Autodesk Fusion 360 part; units mm, degrees
note: some values were not read from the file. Chosen so that the rebuilt part matches the saved one: which bodies a step acts on; a direction. Set by a fixed rule: which sketch regions a step uses.
(part 5 of 5)
sketch "Ear sketch" plane through (0, 0, 0) normal (0, 0, 1) x (1, 0, 0) in component "Stepper bay 28BYJ-48"
  line L0 (-3.4154, 1.0961) -> (0.7978, -2.4393)
  arc A0 (-3.7017, -7.8016) -> (0.7978, -2.4393) centre (-1.4519, -5.1204) ccw
  line L1 (-3.7017, -7.8016) -> (-7.9149, -4.2663)
  arc A1 (-3.4154, 1.0961) -> (-7.9149, -4.2663) centre (-5.6652, -1.5851) ccw
extrude "Ear" add sketch "Ear sketch" along normal blind 7 from surface at 80 bodies 224 in component "Stepper bay 28BYJ-48"
sketch "Ear sketch (1)" plane through (0, 0, 0) normal (0, 0, 1) x (1, 0, 0) in component "Stepper bay 28BYJ-48"
  line L0 (-26.3, 11.1607) -> (-30.5132, 14.696)
  arc A0 (-26.0137, 20.0583) -> (-30.5132, 14.696) centre (-28.2635, 17.3771) ccw
  line L1 (-26.0137, 20.0583) -> (-21.8005, 16.523)
  arc A1 (-26.3, 11.1607) -> (-21.8005, 16.523) centre (-24.0502, 13.8418) ccw
extrude "Ear (1)" add sketch "Ear sketch (1)" along normal blind 7 from surface at 80 bodies 224 in component "Stepper bay 28BYJ-48"
sketch "Wire block sketch" plane through (0, 0, 0) normal (0, 0, 1) x (1, 0, 0) in component "Stepper bay 28BYJ-48"
  line L0 (-9.5224, 23.8435) -> (-12.7364, 20.0132)
  line L1 (-12.7364, 20.0132) -> (-1.5521, 10.6285)
  line L2 (-1.5521, 10.6285) -> (1.6618, 14.4588)
  line L3 (1.6618, 14.4588) -> (-9.5224, 23.8435)
extrude "Wire block" add sketch "Wire block sketch" along normal blind 19 from surface at 68 bodies 224 in component "Stepper bay 28BYJ-48"
component "Tub" placed x (1, 0, 0) y (0, 1, 0) z (0, 0, 1) at (0, 0, 0)
component "Wheel L" placed x (1, 0, 0) y (0, 1, 0) z (0, 0, 1) at (0, 0, 0)
component "Motor L" placed x (1, 0, 0) y (0, 1, 0) z (0, 0, 1) at (0, 0, 0)
component "Wheel R" placed x (1, 0, 0) y (0, 1, 0) z (0, 0, 1) at (0, 0, 0)
component "Motor R" placed x (1, 0, 0) y (0, 1, 0) z (0, 0, 1) at (0, 0, 0)
component "Face plate L" placed x (1, 0, 0) y (0, 1, 0) z (0, 0, 1) at (0, 0, 0)
component "Face plate R" placed x (1, 0, 0) y (0, 1, 0) z (0, 0, 1) at (0, 0, 0)
component "Omni wheel" placed x (1, 0, 0) y (0, 1, 0) z (0, 0, 1) at (0, 0, 0)
component "Omni arm" placed x (1, 0, 0) y (0, 1, 0) z (0, 0, 1) at (0, 0, 0)
component "Omni pins" placed x (1, 0, 0) y (0, 1, 0) z (0, 0, 1) at (0, 0, 0)
component "Omni pivot" placed x (1, 0, 0) y (0, 1, 0) z (0, 0, 1) at (0, 0, 0)
component "Omni spring" placed x (1, 0, 0) y (0, 1, 0) z (0, 0, 1) at (0, 0, 0)
component "Omni adjuster" placed x (1, 0, 0) y (0, 1, 0) z (0, 0, 1) at (0, 0, 0)
component "Rear nub" placed x (1, 0, 0) y (0, 1, 0) z (0, 0, 1) at (0, 0, 0)
component "Bumper L" placed x (1, 0, 0) y (0, 1, 0) z (0, 0, 1) at (0, 0, 0)
component "Bumper switch L" placed x (1, 0, 0) y (0, 1, 0) z (0, 0, 1) at (0, 0, 0)
component "Bumper R" placed x (1, 0, 0) y (0, 1, 0) z (0, 0, 1) at (0, 0, 0)
component "Bumper switch R" placed x (1, 0, 0) y (0, 1, 0) z (0, 0, 1) at (0, 0, 0)
component "Upper frame" placed x (1, 0, 0) y (0, 1, 0) z (0, 0, 1) at (0, 0, 0)
component "ToF F" placed x (1, 0, 0) y (0, 1, 0) z (0, 0, 1) at (0, 0, 0)
component "ToF FL" placed x (1, 0, 0) y (0, 1, 0) z (0, 0, 1) at (0, 0, 0)
component "ToF FR" placed x (1, 0, 0) y (0, 1, 0) z (0, 0, 1) at (0, 0, 0)
component "ToF SFL" placed x (1, 0, 0) y (0, 1, 0) z (0, 0, 1) at (0, 0, 0)
component "ToF SFR" placed x (1, 0, 0) y (0, 1, 0) z (0, 0, 1) at (0, 0, 0)
component "ToF SRL" placed x (1, 0, 0) y (0, 1, 0) z (0, 0, 1) at (0, 0, 0)
component "ToF SRR" placed x (1, 0, 0) y (0, 1, 0) z (0, 0, 1) at (0, 0, 0)
component "ToF RL" placed x (1, 0, 0) y (0, 1, 0) z (0, 0, 1) at (0, 0, 0)
component "ToF RR" placed x (1, 0, 0) y (0, 1, 0) z (0, 0, 1) at (0, 0, 0)
component "Camera L" placed x (1, 0, 0) y (0, 0.34202, 0.939693) z (0, -0.939693, 0.34202) at (3.0712, 87.9464, 93)
component "Camera cage L" placed x (1, 0, 0) y (0, 1, 0) z (0, 0, 1) at (0, 0, 0)
component "Camera R" placed x (-1, 0, 0) y (0, -0.34202, 0.939693) z (0, 0.939693, 0.34202) at (3.0712, -87.9464, 93)
component "Camera cage R" placed x (1, 0, 0) y (0, 1, 0) z (0, 0, 1) at (0, 0, 0)
component "Lid" placed x (1, 0, 0) y (0, 1, 0) z (0, 0, 1) at (0, 0, 0)
component "Handle bar" placed x (1, 0, 0) y (0, 1, 0) z (0, 0, 1) at (0, 0, 0)
component "Victim LED" placed x (1, 0, 0) y (0, 1, 0) z (0, 0, 1) at (0, 0, 0)
component "Start button" placed x (1, 0, 0) y (0, 1, 0) z (0, 0, 1) at (0, 0, 0)
component "Power switch" placed x (1, 0, 0) y (0, 1, 0) z (0, 0, 1) at (0, 0, 0)
component "Status LED 1" placed x (1, 0, 0) y (0, 1, 0) z (0, 0, 1) at (0, 0, 0)
component "Status LED 2" placed x (1, 0, 0) y (0, 1, 0) z (0, 0, 1) at (0, 0, 0)
component "USB-C service socket" placed x (1, 0, 0) y (0, 1, 0) z (0, 0, 1) at (0, 0, 0)
component "Dropper floor" placed x (1, 0, 0) y (0, 1, 0) z (0, 0, 1) at (0, 0, 0)
component "Dropper plate" placed x (1, 0, 0) y (0, 1, 0) z (0, 0, 1) at (0, 0, 0)
component "N20 motor" placed x (1, 0, 0) y (0, 1, 0) z (0, 0, 1) at (0, 0, 0)
component "N20 face plate" placed x (1, 0, 0) y (0, 1, 0) z (0, 0, 1) at (0, 0, 0)
component "Kits" placed x (1, 0, 0) y (0, 1, 0) z (0, 0, 1) at (0, 0, 0)
component "Hopper B left" placed x (1, 0, 0) y (0, 1, 0) z (0, 0, 1) at (0, 0, 0)
component "Chute B left" placed x (1, 0, 0) y (0, 1, 0) z (0, 0, 1) at (0, 0, 0)
component "Hopper A right" placed x (1, 0, 0) y (0, 1, 0) z (0, 0, 1) at (0, 0, 0)
component "Chute A right" placed x (1, 0, 0) y (0, 1, 0) z (0, 0, 1) at (0, 0, 0)
component "GIGA posts" placed x (1, 0, 0) y (0, 1, 0) z (0, 0, 1) at (0, 0, 0)
component "Arduino GIGA R1" placed x (1, 0, 0) y (0, 1, 0) z (0, 0, 1) at (0, 0, 0)
component "Main PCB" placed x (1, 0, 0) y (0, 1, 0) z (0, 0, 1) at (0, 0, 0)
component "Battery" placed x (1, 0, 0) y (0, 1, 0) z (0, 0, 1) at (0, 0, 0)
component "Floor port FP" placed x (1, 0, 0) y (0, 1, 0) z (0, 0, 1) at (0, 0, 0)
component "Silver module SM" placed x (1, 0, 0) y (0, 1, 0) z (0, 0, 1) at (0, 0, 0)
component "Wi-Fi antenna" placed x (1, 0, 0) y (0, 1, 0) z (0, 0, 1) at (0, 0, 0)
component "BNO055 IMU" placed x (1, 0, 0) y (0, 1, 0) z (0, 0, 1) at (0, 0, 0)
component "Stepper bay 28BYJ-48" placed x (1, 0, 0) y (0, 1, 0) z (0, 0, 1) at (0, 0, 0)
named bodies: "Tub shell", "Chute hole tool B left", "Chute hole tool A right", "Cradle prong front L", "Cradle prong rear L", "Cradle prong front R", "Cradle prong rear R", "Wheel L", "Encoder L", "Gearmotor L", "Motor shaft L", "Wheel R", "Encoder R", "Gearmotor R", "Motor shaft R", "Face plate L", "Face plate R", "Omni wheel", "Bearing inboard", "Bearing outboard", "Axle sleeve", "Axle spacer", "Arm bar", "Seat pin", "Spring forward leg", "Axle screw", "Axle screw head", "Axle washer", "Pivot screw", "Pivot screw head", "Stop screw", "Stop screw head", "Pivot tube", "Spring coil", "Spring rear leg", "Spring arbor", "Adjuster screw head", "Adjuster screw", "Rear nub", "Bumper plate L", "Microswitch L", "Bumper plate R", "Microswitch R", "Frame ring", "VL53L0X board F", "QT connector F", "QT connector F (1)", "VL53L0X chip F", "M2.5 screw heads F 1", "M2.5 screw heads F 2", "M2.5 screw shafts F 1", "M2.5 screw shafts F 2", "VL53L0X board FL", "QT connector FL", "QT connector FL (1)", "VL53L0X chip FL", "M2.5 screw heads FL 1", "M2.5 screw heads FL 2", "M2.5 screw shafts FL 1", "M2.5 screw shafts FL 2", "VL53L0X board FR", "QT connector FR", "QT connector FR (1)", "VL53L0X chip FR", "M2.5 screw heads FR 1", "M2.5 screw heads FR 2", "M2.5 screw shafts FR 1", "M2.5 screw shafts FR 2", "VL53L0X board SFL", "QT connector SFL", "QT connector SFL (1)", "VL53L0X chip SFL", "M2.5 screw heads SFL 1", "M2.5 screw heads SFL 2", "M2.5 screw shafts SFL 1", "M2.5 screw shafts SFL 2", "VL53L0X board SFR", "QT connector SFR", "QT connector SFR (1)", "VL53L0X chip SFR", "M2.5 screw heads SFR 1", "M2.5 screw heads SFR 2", "M2.5 screw shafts SFR 1", "M2.5 screw shafts SFR 2", "VL53L0X board SRL", "QT connector SRL", "QT connector SRL (1)", "VL53L0X chip SRL", "M2.5 screw heads SRL 1", "M2.5 screw heads SRL 2", "M2.5 screw shafts SRL 1", "M2.5 screw shafts SRL 2", "VL53L0X board SRR", "QT connector SRR", "QT connector SRR (1)", "VL53L0X chip SRR", "M2.5 screw heads SRR 1", "M2.5 screw heads SRR 2", "M2.5 screw shafts SRR 1", "M2.5 screw shafts SRR 2", "VL53L0X board RL", "QT connector RL", "QT connector RL (1)", "VL53L0X chip RL", "M2.5 screw heads RL 1", "M2.5 screw heads RL 2", "M2.5 screw shafts RL 1", "M2.5 screw shafts RL 2", "VL53L0X board RR", "QT connector RR", "QT connector RR (1)", "VL53L0X chip RR", "M2.5 screw heads RR 1", "M2.5 screw heads RR 2", "M2.5 screw shafts RR 1", "M2.5 screw shafts RR 2", "OpenMV H7 Plus board L", "Lens holder L", "Lens barrel L", "micro-SD socket L", "M2.5 screw heads L 1", "M2.5 screw heads L 2", "M2.5 screw heads L 3", "M2.5 screw heads L 4", "M2.5 screw shafts L 1", "M2.5 screw shafts L 2", "M2.5 screw shafts L 3", "M2.5 screw shafts L 4", "Cage frame L", "Cage rails L 1", "Cage rails L 2", "Cage flange L", "Cage barrel opening L", "Cage pilots L 1", "Cage pilots L 2", "Cage pilots L 3", "Cage pilots L 4", "Cage ears L 1", "Cage ears L 2", "OpenMV H7 Plus board R", "Lens holder R", "Lens barrel R", "micro-SD socket R", "M2.5 screw heads R 1", "M2.5 screw heads R 2", "M2.5 screw heads R 3", "M2.5 screw heads R 4", "M2.5 screw shafts R 1", "M2.5 screw shafts R 2", "M2.5 screw shafts R 3", "M2.5 screw shafts R 4", "Cage frame R", "Cage rails R 1", "Cage rails R 2", "Cage flange R", "Cage barrel opening R", "Cage pilots R 1", "Cage pilots R 2", "Cage pilots R 3", "Cage pilots R 4", "Cage ears R 1", "Cage ears R 2", "Lid plate", "Hook bump +71", "Hook bump +114", "Hook bump -71", "Hook bump -114", "Handle bar", "Victim LED", "Start button", "Power switch", "Status LED 1", "Status LED 2", "USB-C service socket", "Dropper floor", "Dropper plate", "N20 gearmotor with encoder", "N20 shaft", "N20 face plate", "Kit 1", "Kit 2", "Kit 3", "Kit 4", "Kit 5", "Kit 6", "Kit 7", "Kit 8", "Hopper", "Socket tool", "Channel", "Channel void", "Floor slab", "Trim", "GIGA post H1", "GIGA post H2", "GIGA post H3", "GIGA post H4", "GIGA board", "Header strip +y", "Header strip -y", "Main PCB shield (placeholder)", "PCB component envelope (placeholder)", "Battery (placeholder 7.0 x 3.5 x 2.5)", "Floor sensor FP (black, blue, red)", "Silver module SM (straight + 20 deg tilted pair)", "USB-C J12", "Wi-Fi antenna", "BNO055 board", "BNO055 chip", "M2.5 screw heads 1", "M2.5 screw heads 2", "M2.5 screw heads 3", "M2.5 screw heads 4", "M2.5 screw shafts 1", "M2.5 screw shafts 2", "M2.5 screw shafts 3", "M2.5 screw shafts 4", "Body"
